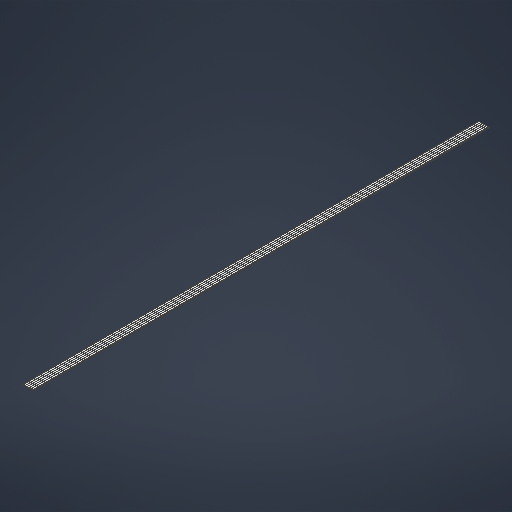
# Autodesk Inventor part: SP40-12 REVESTIMIENTO - TABLILLA
Saved by Autodesk Inventor 2025 (Build 290162000, 162)
## iProperties
Created: 2026-01-30
Part Number: SP40-12 REVESTIMIENTO - TABLILLA
Material: Aluminio
Document SubType Name: Modeling
Designer: ROLANDO
Density: 2.7 g/cm^3
Appearance: Satinado
Author: ROLANDO
Autodesk Inventor part; units mm, degrees
ref_plane "YZ Plane" through (0, 0, 0) normal (1, 0, 0) x (0, 1, 0)
ref_plane "XZ Plane" through (0, 0, 0) normal (0, 1, 0) x (-1, 0, 0)
ref_plane "XY Plane" through (0, 0, 0) normal (0, 0, 1) x (1, 0, 0)
sketch "Boceto1" plane through (0, 0, 0) normal (0, 0, 1) x (1, 0, 0)
  line L0 (0, 7) -> (114.5, 7)
  line L1 (114.5, 0) -> (0, 0)
  line L2 (0, 1.8) -> (-1.7033, 1.8)
  line L3 (0, 5.2) -> (-1.7033, 5.2)
  line L4 (-15.7075, 3.5) -> (143.059, 3.5) construction
  line L5 (20.7, 5.065) -> (20.7, 1.935)
  line L6 (22, 5.065) -> (22, 1.935)
  line L7 (41.4, 5.065) -> (41.4, 1.935)
  line L8 (-4.39, 1.4) -> (-4.9501, 1.87)
  line L9 (-4.9501, 1.87) -> (-4.9501, 2.4)
  line L10 (20.04, 5.7) -> (1.3, 5.7)
  line L11 (1.3, 1.3) -> (20.04, 1.3)
  line L12 (22.66, 1.3) -> (40.74, 1.3)
  line L13 (40.74, 5.7) -> (22.66, 5.7)
  line L14 (114.5, 7) -> (114.5, 5.8)
  line L15 (114.5, 1.2) -> (114.5, 0)
  line L16 (-1.7033, 1.8) -> (-2.18, 1.4)
  line L17 (-2.18, 1.4) -> (-4.39, 1.4)
  line L18 (-1.7033, 5.2) -> (-2.18, 5.6)
  line L19 (-4.9501, 4.6) -> (-2.544, 4.6)
  line L20 (-4.9501, 2.4) -> (-2.544, 2.4)
  line L21 (-2.544, 2.4) -> (-1.6895, 3.117)
  line L22 (-2.544, 4.6) -> (-1.6895, 3.883)
  line L23 (0, 0) -> (0, 1.8)
  line L24 (0, 5.2) -> (0, 7)
  line L25 (-0.1237, 3.933) -> (1.3, 4.755)
  line L26 (-0.1237, 3.067) -> (1.3, 2.245)
  line L27 (1.3, 5.7) -> (1.3, 4.755)
  line L28 (1.3, 2.245) -> (1.3, 1.3)
  line L29 (-4.9501, 5.13) -> (-4.39, 5.6)
  line L30 (-2.18, 5.6) -> (-4.39, 5.6)
  line L31 (-4.9501, 4.6) -> (-4.9501, 5.13)
  arc A0 (-0.1237, 3.933) -> (-0.1237, 3.067) centre (0.1263, 3.5) ccw
  arc A1 (-1.6895, 3.117) -> (-1.6895, 3.883) centre (-2.0109, 3.5) ccw
  line L32 (20.04, 5.7) -> (20.7, 5.065)
  line L33 (20.04, 1.3) -> (20.7, 1.935)
  line L34 (22, 5.065) -> (22.66, 5.7)
  line L35 (22, 1.935) -> (22.66, 1.3)
  line L36 (40.74, 5.7) -> (41.4, 5.065)
  line L37 (40.74, 1.3) -> (41.4, 1.935)
  line L38 (61.44, 1.3) -> (62.1, 1.935)
  line L39 (62.1, 5.065) -> (62.1, 1.935)
  line L40 (61.44, 5.7) -> (62.1, 5.065)
  line L41 (42.7, 5.065) -> (42.7, 1.935)
  line L42 (43.36, 1.3) -> (61.44, 1.3)
  line L43 (61.44, 5.7) -> (43.36, 5.7)
  line L44 (42.7, 5.065) -> (43.36, 5.7)
  line L45 (42.7, 1.935) -> (43.36, 1.3)
  line L46 (82.14, 1.3) -> (82.8, 1.935)
  line L47 (82.8, 5.065) -> (82.8, 1.935)
  line L48 (82.14, 5.7) -> (82.8, 5.065)
  line L49 (63.4, 5.065) -> (63.4, 1.935)
  line L50 (64.06, 1.3) -> (82.14, 1.3)
  line L51 (82.14, 5.7) -> (64.06, 5.7)
  line L52 (63.4, 5.065) -> (64.06, 5.7)
  line L53 (63.4, 1.935) -> (64.06, 1.3)
  line L54 (102.84, 1.3) -> (103.5, 1.935)
  line L55 (103.5, 5.065) -> (103.5, 1.935)
  line L56 (102.84, 5.7) -> (103.5, 5.065)
  line L57 (84.1, 5.065) -> (84.1, 1.935)
  line L58 (84.76, 1.3) -> (102.84, 1.3)
  line L59 (102.84, 5.7) -> (84.76, 5.7)
  line L60 (84.1, 5.065) -> (84.76, 5.7)
  line L61 (84.1, 1.935) -> (84.76, 1.3)
  line L62 (104.8, 5.065) -> (105.46, 5.7)
  line L63 (104.8, 5.065) -> (104.8, 1.935)
  line L64 (104.8, 1.935) -> (105.46, 1.3)
  line L65 (105.46, 5.7) -> (112.5, 5.7)
  line L66 (105.46, 1.3) -> (112.5, 1.3)
  line L67 (112.5, 5.7) -> (112.9, 5.3)
  line L68 (112.9, 5.3) -> (114, 5.3)
  line L69 (114, 5.3) -> (114.5, 5.8)
  line L70 (112.5, 1.3) -> (112.9, 1.7)
  line L71 (112.9, 1.7) -> (114, 1.7)
  line L72 (114, 1.7) -> (114.5, 1.2)
  point P0 (-1.233, 3.5)
  point P1 (-0.8737, 3.5)
  dimension "d4" = 7
  dimension "d9" = 3.4
  dimension "d11" = 2.1
  dimension "d12" = 1
  dimension "d13" = 1
  dimension "d14" = 1
  dimension "d22" = 1.3
  dimension "d25" = 1.3
  dimension "d26" = 1.3
  dimension "d27" = 30
  dimension "d28" = 60
  dimension "d29" = 1.255
  dimension "d30" = 2.51
  dimension "d33" = 1.3
  dimension "d34" = 3.5
  dimension "d37" = 1.3
  dimension "d42" = 2.18
  dimension "d46" = 50
  dimension "d47" = 50
  dimension "d50" = 4.2
  dimension "d52" = 1
  dimension "d53" = 0.47
  dimension "d54" = 0.47
  dimension "d57" = 4.39
  dimension "d61" = 1.7
  dimension "d62" = 3.5
  dimension "d65" = 0.5
  dimension "d66" = 0.5
  dimension "d67" = 19.4
  dimension "d68" = 0.66
  dimension "d69" = 0.66
  dimension "d70" = 1.565
  dimension "d71" = 3.13
  dimension "d73" = 19.4
  dimension "d74" = 0.66
  dimension "d75" = 1.565
  dimension "d78" = 0.66
  dimension "d80" = 3.13
  dimension "d81" = 0.66
  dimension "d82" = 0.66
  dimension "d83" = 1.565
  dimension "d84" = 3.13
  dimension "d87" = 20.7
  dimension "d94" = 20.7
  dimension "d99" = 2.3
  dimension "d100" = 4.6
  dimension "d101" = 1.8
  dimension "d102" = 3.6
  dimension "d103" = 4.4
  dimension "d104" = 4.4
  dimension "d105" = 2
  dimension "d106" = 2
  dimension "d107" = 45
  dimension "d109" = 90
  dimension "d110" = 90
  dimension "d111" = 114.5
  dimension "d112" = 119.4501
  constraints: 146 end point, 18 parallel, 14 horizontal, 8 perpendicular, 6 collinear, 6 point on line, 4 point on circle, 4 tangent, 3 equal length, 2 centre point, 1 coincident, 1 vertical, 54 other
  measures "d4" distance between parallel lines of L1 L0
  measures "d9" distance between parallel lines of L2 L3
  measures "d11" distance between parallel lines of L4 L17
  measures "d12" distance between parallel lines of L21 L16
  measures "d13" distance between parallel lines of L18 L22
  measures "d14" distance between parallel lines of L17 L20
  measures "d22" distance between parallel lines of L6 L5
  measures "d25" distance between parallel lines of L24 L27
  measures "d26" distance between parallel lines of L28 L23
  measures "d27" angle of L4 L25
  measures "d28" angle of L25 L26
  measures "d29" distance from line of L4 L25.end
  measures "d30" distance of L25.end L26.end
  measures "d33" distance between parallel lines of L1 L11
  measures "d34" distance between parallel lines of L1 L4
  measures "d37" distance between parallel lines of L10 L0
  measures "d42" distance from line of L23 L16.end
  measures "d46" angle of L23 L16
  measures "d47" angle of L24 L18
  measures "d50" distance between parallel lines of L17 L30
  measures "d52" distance between parallel lines of L30 L19
  measures "d53" vertical distance of L29.start L29.end
  measures "d54" vertical distance of L8.start L8.end
  measures "d57" distance from line of L24 L29.end
  measures "d61" distance between parallel lines of L4 L2
  measures "d62" distance between parallel lines of L0 L4
  measures "d65" radius of A0
  measures "d66" radius of A1
  measures "d67" distance from line of L25.end L5
  measures "d68" horizontal distance of L10.start L5.start
  measures "d69" horizontal distance of L11.end L5.end
  measures "d70" distance from line of L5.start L4
  measures "d71" distance of L5.end L5.start
  measures "d73" distance between parallel lines of L7 L6
  measures "d74" horizontal distance of L6.start L13.end
  measures "d75" distance from line of L6.start L4
  measures "d78" horizontal distance of L12.start L6.end
  measures "d80" distance of L6.start L6.end
  measures "d81" horizontal distance of L13.start L7.start
  measures "d82" horizontal distance of L12.end L7.end
  measures "d83" distance from line of L7.start L4
  measures "d84" distance of L7.start L7.end
  measures "d87" distance of L12.end L38.start
  measures "d94" distance of L57.start L62.start
  measures "d99" distance from line of L4 L14.end
  measures "d100" distance of L15.start L14.end
  measures "d101" distance between parallel lines of L4 L68
  measures "d102" distance between parallel lines of L71 L68
  measures "d103" distance between parallel lines of L11 L10
  measures "d104" distance between parallel lines of L66 L65
  measures "d105" horizontal distance of L15.start L66.end
  measures "d106" horizontal distance of L14.end L65.end
  measures "d107" angle of L4 L69
  measures "d109" angle of L69 L72
  measures "d110" angle of L72 L70
  measures "d111" distance between parallel lines of L15 L23
  measures "d112" distance between parallel lines of L15 L9
extrude "Extrusión1" add sketch "Boceto1" against normal blind 5000
